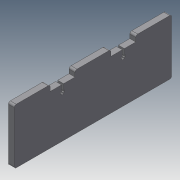
# Autodesk Inventor part: InnerSide
Saved by Autodesk Inventor 2014 (Build 180170000, 170)
## iProperties
Created: 2015-01-19
Part Number: InnerSide
Material: Generic
Document SubType Name: Modeling
Designer: Peele
Density: 1 g/cm^3
Appearance: Default
Author: Peele
Autodesk Inventor part; units mm, degrees
ref_plane "YZ Plane" through (0, 0, 0) normal (1, 0, 0) x (0, 1, 0)
ref_plane "XZ Plane" through (0, 0, 0) normal (0, 1, 0) x (-1, 0, 0)
ref_plane "XY Plane" through (0, 0, 0) normal (0, 0, 1) x (1, 0, 0)
sketch "Sketch1" plane through (0, 0, 0) normal (1, 0, 0) x (0, 1, 0)
  line L0 (80, -25) -> (-80, -25)
  line L1 (-80, -25) -> (-80, 25)
  line L2 (-80, 25) -> (80, 25)
  line L3 (80, 25) -> (80, -25)
  line L4 (80, -25) -> (-80, 25) construction
  line L5 (-80, -25) -> (80, 25) construction
  point P0 (0, 0)
  dimension "d0" = 160
  dimension "d1" = 50
  constraints: 12 end point, 2 midpoint, 2 parallel, 1 horizontal, 1 perpendicular
  measures "d0" distance of L1.end L2.end
  measures "d1" distance of L2.end L0.start
extrude "Extrusion1" add sketch "Sketch1" along normal blind 6
sketch "Sketch2" plane through (6, 0, 0) normal (1, 0, 0) x (0, 0, -1)
  line L0 (-25, 80) -> (-25, -80) projected
  line L1 (-25, 80) -> (-31, 80)
  line L2 (-31, 80) -> (-31, 43.5)
  line L3 (-31, 43.5) -> (-25, 43.5)
  line L4 (-25, 43.5) -> (-25, 80)
  line L5 (-25, 18.25) -> (-31, 18.25)
  line L6 (-31, 18.25) -> (-31, -18.25)
  line L7 (-31, -18.25) -> (-25, -18.25)
  line L8 (-25, -18.25) -> (-25, 18.25)
  line L9 (-25, -80) -> (-31, -80)
  line L10 (-31, -80) -> (-31, -43.5)
  line L11 (-31, -43.5) -> (-25, -43.5)
  line L12 (-25, -43.5) -> (-25, -80)
  point P0 (0, 0)
  dimension "d4" = 6
  dimension "d5" = 25.25
  dimension "d6" = 25.25
  constraints: 24 end point, 6 parallel, 4 collinear, 3 horizontal, 3 perpendicular, 1 point on line
  measures "d4" distance of L0.start L1.end
  measures "d5" distance between parallel lines of L5 L3
  measures "d6" distance between parallel lines of L11 L7
extrude "Extrusion2" add sketch "Sketch2" against normal blind 6
sketch "Sketch3" plane through (6, 0, 0) normal (1, 0, 0) x (0, 0, -1)
  line L0 (-25, 43.5) -> (-25, 18.25) projected
  line L1 (-31, -80) -> (25, -80) projected
  line L2 (-25, 30.875) -> (0, 30.875) construction
  line L3 (-25, 29.825) -> (-25, 31.925)
  line L4 (-25, 31.925) -> (-19, 31.925)
  line L5 (-19, 31.925) -> (-19, 32.925)
  line L6 (-19, 32.925) -> (-17.2, 32.925)
  line L7 (-17.2, 32.925) -> (-17.2, 31.925)
  line L8 (-17.2, 31.925) -> (-16, 31.925)
  line L9 (-16, 31.925) -> (-16, 29.825)
  line L10 (-16, 29.825) -> (-17.2, 29.825)
  line L11 (-17.2, 29.825) -> (-17.2, 28.825)
  line L12 (-17.2, 28.825) -> (-19, 28.825)
  line L13 (-19, 28.825) -> (-19, 29.825)
  line L14 (-19, 29.825) -> (-25, 29.825)
  point P0 (0, 0)
  dimension "d9" = 1.8
  dimension "d10" = 4.1
  dimension "d11" = 2.1
  dimension "d12" = 1.05
  dimension "d13" = 9
  dimension "d14" = 2.05
  dimension "d15" = 6
  constraints: 26 end point, 8 parallel, 6 collinear, 2 perpendicular, 2 point on line, 1 midpoint
  measures "d9" distance of L5.end L6.end
  measures "d10" distance between parallel lines of L6 L12
  measures "d11" distance between parallel lines of L14 L4
  measures "d12" distance between parallel lines of L4 L2
  measures "d13" distance between parallel lines of L0 L9
  measures "d14" distance between parallel lines of L6 L2
  measures "d15" distance between parallel lines of L0 L5
extrude "Extrusion3" cut sketch "Sketch3" against normal through all
mirror "Mirror1" about plane through (0, 0, 0) normal (0, 1, 0) of "Extrusion3"
fillet "Fillet1" radius 2 8 edges at (3, 43.5, 31) (3, 80, 31) (3, 18.25, 31) (3, -18.25, 31) (3, -43.5, 31) (3, -80, 31) (3, 80, -25) (3, -80, -25)
equation "\"d12\" = 0.5 * d11"
equation "\"d14\" = 0.5 * d10"
body "Solid1"
